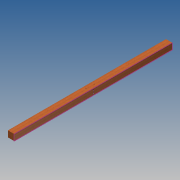
# Autodesk Inventor part: hubjig_side1
Saved by Autodesk Inventor 2014 SP1 (Build 180222100, 222)
## iProperties
Created: 2014-08-29
Part Number: hubjig_side1
Material: Wood (Cherry)
Document SubType Name: Modeling
Designer: Dave
Mass: 2168.01 g
Surface Area: 2648.38 cm^2
Volume: 3441.28 cm^3
Density: 0.63 g/cm^3
Appearance: Cherry - Natural Low Gloss
Author: Dave
Autodesk Inventor part; units mm, degrees
ref_plane "YZ Plane" through (0, 0, 0) normal (1, 0, 0) x (0, 1, 0)
ref_plane "XZ Plane" through (0, 0, 0) normal (0, 1, 0) x (-1, 0, 0)
ref_plane "XY Plane" through (0, 0, 0) normal (0, 0, 1) x (1, 0, 0)
sketch "Sketch1" plane through (0, 0, 0) normal (0, 0, 1) x (1, 0, 0)
  line L0 (0, 0) -> (38.1, 0)
  line L1 (38.1, 0) -> (38.1, 38.1)
  line L2 (38.1, 38.1) -> (0, 38.1)
  line L3 (0, 38.1) -> (0, 0)
  dimension "d0" = 38.1
  dimension "d1" = 38.1
  constraints: 8 end point, 2 parallel, 1 horizontal, 1 perpendicular
  measures "d0" distance of L0.start L0.end
  measures "d1" distance of L2.end L0.start
extrude "Extrusion1" add sketch "Sketch1" along normal blind 990.6
sketch "Sketch3" plane through (0, 38.1, 0) normal (0, 1, 0) x (1, 0, 0)
  line L0 (0, 0) -> (0, -990.6) projected
  line L1 (38.1, 0) -> (38.1, -990.6) projected
  line L2 (0, -495.3) -> (38.1, -495.3) construction
  circle A0 centre (19.05, -469.9) radius 4.1388
  circle A1 centre (19.05, -520.7) radius 4.1388
  dimension "d21" = 25.4
  constraints: 2 centre point, 2 end point, 2 midpoint, 1 symmetric about line, 1 other
  measures "d21" distance from line of L2 A0.centre
hole "Hole2" at (19.05, 38.1, 469.9) at (19.05, 38.1, 520.7) direction (0, -1, 0) diameter 5.1054 depth 25.4 tip angle 118 clearance for "Flat Head Machine Screw (82)" size "#10" standard "Ansi Unified Screw Threads"
sketch "Sketch4" plane through (38.1, 0, 0) normal (1, 0, 0) x (0, 0, -1)
  line L0 (0, 0) -> (0, 38.1) projected
  line L1 (0, 38.1) -> (-990.6, 38.1) projected
  line L2 (-990.6, 0) -> (-990.6, 38.1) projected
  line L3 (0, 0) -> (-990.6, 0) projected
  line L4 (-495.3, 38.1) -> (-495.3, 0) construction
  constraints: 2 end point, 2 midpoint
body "Solid1"
